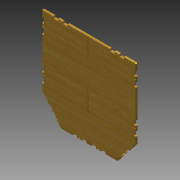
# Autodesk Inventor part: tampa_mdf
Saved by Autodesk Inventor 2014 (Build 180170000, 170)
## iProperties
Created: 2014-11-10
Part Number: tampa_mdf
Material: Generic
Document SubType Name: Modeling
Designer: Gabriel
Density: 1 g/cm^3
Appearance: Default
Author: Gabriel
Autodesk Inventor part; units mm, degrees
ref_plane "YZ Plane" through (0, 0, 0) normal (1, 0, 0) x (0, 1, 0)
ref_plane "XZ Plane" through (0, 0, 0) normal (0, 1, 0) x (-1, 0, 0)
ref_plane "XY Plane" through (0, 0, 0) normal (0, 0, 1) x (1, 0, 0)
sketch "Sketch1" plane through (0, 0, 0) normal (0, 1, 0) x (-1, 0, 0)
  line L0 (0, -150) -> (40, -200)
  line L1 (160, -200) -> (200, -150)
  line L2 (0, -150) -> (0, -120)
  line L3 (0, -150) -> (0, -120)
  line L4 (0, -120) -> (0, -150)
  line L5 (200, -120) -> (200, -150)
  line L6 (40, -200) -> (65, -200)
  line L7 (160, -200) -> (135, -200)
  line L8 (65, -200) -> (40, -200)
  line L9 (200, -120) -> (200, -150)
  line L10 (0, -120) -> (0, 0)
  line L11 (200, 0) -> (200, -120)
  line L12 (0, 0) -> (200, 0)
  line L13 (0, 0) -> (2.5, 0)
  line L14 (65, -200) -> (135, -200)
  line L15 (160, -200) -> (169.9951, -187.5061)
  line L16 (169.9951, -187.5061) -> (189.9854, -162.5183)
  line L17 (189.9854, -162.5183) -> (188.0332, -160.9566)
  circle A0 centre (188.0332, -160.9566) radius 1.5
  circle A1 centre (168.0429, -185.9444) radius 1.5
  line L18 (40, -200) -> (30.0049, -187.5061)
  line L19 (30.0049, -187.5061) -> (31.9571, -185.9444)
  circle A2 centre (31.9571, -185.9444) radius 1.5
  circle A3 centre (11.9668, -160.9566) radius 1.5
  line L20 (40, -200) -> (33.753, -192.1913)
  line L21 (27.5061, -184.3826) -> (21.2591, -176.5739)
  line L22 (0, -150) -> (6.247, -157.8087)
  line L23 (12.4939, -165.6174) -> (18.7409, -173.4261)
  line L24 (160, -200) -> (166.247, -192.1913)
  line L25 (166.247, -192.1913) -> (172.4939, -184.3826)
  line L26 (168.98, -184.7731) -> (168.0429, -185.9444)
  line L27 (200, -150) -> (193.753, -157.8087)
  line L28 (193.753, -157.8087) -> (187.5061, -165.6174)
  line L29 (187.5061, -165.6174) -> (181.2591, -173.4261)
  line L30 (135, -200) -> (135, -195)
  line L31 (135, -195) -> (125, -195)
  line L32 (125, -195) -> (125, -200)
  line L33 (125, -195) -> (115, -195)
  line L34 (115, -195) -> (115, -200)
  line L35 (115, -195) -> (105, -195)
  line L36 (105, -195) -> (105, -200)
  line L37 (40, -200) -> (65, -200)
  line L38 (65, -200) -> (65, -195)
  line L39 (65, -195) -> (75, -195)
  line L40 (75, -195) -> (75, -200)
  line L41 (75, -200) -> (85, -200)
  line L42 (85, -200) -> (85, -195)
  line L43 (85, -195) -> (95, -195)
  line L44 (95, -195) -> (95, -200)
  line L45 (0, -150) -> (0, -105)
  line L46 (0, -95) -> (0, -85)
  line L47 (0, -75) -> (0, -45)
  line L48 (0, -45) -> (5, -45)
  line L49 (5, -45) -> (5, -35)
  line L50 (5, -35) -> (0, -35)
  line L51 (0, -35) -> (0, -25)
  line L52 (0, -25) -> (5, -25)
  line L53 (5, -25) -> (5, -15)
  line L54 (5, -15) -> (0, -15)
  line L55 (0, -45) -> (200, -45)
  line L56 (195, -45) -> (195, -35)
  line L57 (195, -35) -> (200, -35)
  line L58 (0, -25) -> (200, -25)
  line L59 (195, -25) -> (195, -15)
  line L60 (195, -15) -> (200, -15)
  line L61 (0, 0) -> (25, 0)
  line L62 (25, 0) -> (25, -5)
  line L63 (25, -5) -> (35, -5)
  line L64 (35, -5) -> (35, 0)
  line L65 (35, -5) -> (45, -5)
  line L66 (45, -5) -> (45, 0)
  line L67 (45, -5) -> (55, -5)
  line L68 (55, -5) -> (55, 0)
  line L69 (200, 0) -> (175, 0)
  line L70 (175, 0) -> (175, -5)
  line L71 (175, -5) -> (165, -5)
  line L72 (165, -5) -> (165, 0)
  line L73 (165, -5) -> (155, -5)
  line L74 (155, -5) -> (155, 0)
  line L75 (155, -5) -> (145, -5)
  line L76 (145, -5) -> (145, 0)
  line L77 (40, -200) -> (30.0049, -187.5061)
  line L78 (30, -187.5) -> (32.1871, -190.2338)
  line L79 (11.9668, -160.9566) -> (10.0146, -162.5183)
  line L80 (0, -150) -> (10.0146, -162.5183)
  line L81 (10.0146, -162.5183) -> (8.7059, -160.8824)
  line L82 (168.0429, -185.9444) -> (169.9951, -187.5061)
  line L83 (160, -200) -> (169.9951, -187.5061)
  line L84 (169.9951, -187.5061) -> (167.8081, -190.2399)
  line L85 (189.9854, -162.5183) -> (191.2941, -160.8824)
  line L86 (40, -200) -> (39.3753, -199.2191)
  line L87 (30, -187.5) -> (28.4431, -185.5539)
  line L88 (28.4431, -185.5539) -> (30.8818, -183.603)
  line L89 (30.8818, -183.603) -> (24.6348, -175.7943)
  line L90 (24.6348, -175.7943) -> (22.1962, -177.7452)
  line L91 (169.9951, -187.5061) -> (171.5569, -185.5539)
  line L92 (171.5569, -185.5539) -> (169.1182, -183.603)
  line L93 (169.1182, -183.603) -> (175.3652, -175.7943)
  line L94 (175.3652, -175.7943) -> (177.8038, -177.7452)
  line L95 (22.1962, -177.7452) -> (20.5545, -175.6931)
  line L96 (20.5545, -175.6931) -> (22.9931, -173.7422)
  line L97 (22.9931, -173.7422) -> (16.7462, -165.9335)
  line L98 (16.7462, -165.9335) -> (14.3075, -167.8844)
  line L99 (177.8038, -177.7452) -> (179.4455, -175.6931)
  line L100 (179.4455, -175.6931) -> (177.0069, -173.7422)
  line L101 (177.0069, -173.7422) -> (183.2538, -165.9335)
  line L102 (183.2538, -165.9335) -> (185.6925, -167.8844)
  line L103 (0, -45) -> (0, -105)
  line L104 (0, -105) -> (5, -105)
  line L105 (5, -105) -> (5, -115)
  line L106 (5, -115) -> (0, -115)
  line L107 (5, -125) -> (0, -125)
  line L108 (5, -125) -> (5, -135)
  line L109 (5, -135) -> (0, -135)
  line L110 (5, -135) -> (200, -135)
  line L111 (5, -125) -> (200, -125)
  line L112 (5, -115) -> (200, -115)
  line L113 (5, -105) -> (200, -105)
  line L114 (200, -115) -> (195, -115)
  line L115 (195, -115) -> (195, -105)
  line L116 (195, -135) -> (195, -125)
  line L117 (0, -125) -> (0, -120)
  line L118 (0, -120) -> (2.5, -120)
  circle A4 centre (2.5, -120) radius 1.5
  line L119 (200, -120) -> (197.5, -120)
  circle A5 centre (197.5, -120) radius 1.5
  point P0 (200, -95)
  point P1 (200, -85)
  point P2 (200, -75)
  point P3 (33.1284, -191.4104)
  dimension "d293" = 3
  dimension "d2" = 150
  dimension "d6" = 200
  dimension "d26" = 25
  dimension "d37" = 30
  dimension "d41" = 2.5
  dimension "d277" = 120
  dimension "d296" = 16
  dimension "d297" = 32
  dimension "d299" = 3
  dimension "d333" = 10
  dimension "d338" = 10
  dimension "d342" = 10
  dimension "d363" = 5
  dimension "d364" = 10
  dimension "d365" = 10
  dimension "d366" = 10
  dimension "d367" = 25
  dimension "d368" = 5
  dimension "d369" = 10
  dimension "d370" = 10
  dimension "d371" = 10
  dimension "d381" = 5
  dimension "d382" = 10
  dimension "d383" = 10
  dimension "d384" = 5
  dimension "d385" = 10
  dimension "d391" = 25
  dimension "d392" = 5
  dimension "d393" = 10
  dimension "d394" = 10
  dimension "d395" = 10
  dimension "d396" = 25
  dimension "d397" = 5
  dimension "d398" = 10
  dimension "d401" = 10
  dimension "d402" = 10
  dimension "d408" = 2.095
  dimension "d434" = 3.123
  dimension "d435" = 10
  dimension "d436" = 2.5
  dimension "d437" = 2.5
  dimension "d438" = 3.123
  dimension "d439" = 10
  dimension "d440" = 2.628
  dimension "d441" = 3.123
  dimension "d442" = 10
  dimension "d443" = 2.628
  dimension "d444" = 3.123
  dimension "d445" = 10
  dimension "d448" = 20
  dimension "d449" = 60
  dimension "d450" = 5
  dimension "d451" = 10
  dimension "d453" = 10
  dimension "d454" = 10
  dimension "d455" = 5
  dimension "d456" = 10
  dimension "d459" = 5
  dimension "d460" = 2.5
  dimension "d461" = 3
  dimension "d462" = 2.5
  dimension "d463" = 3
  constraints: 232 end point, 41 perpendicular, 38 point on line, 10 parallel, 8 horizontal, 8 vertical, 7 coincident, 5 centre point, 5 collinear, 1 midpoint, 57 other
  measures "d2" distance of L2.start point (0, 0)
  measures "d6" distance of L1.end L2.start
  measures "d26" distance of L1.start L7.end
  measures "d37" distance of L5.start L1.end
  measures "d41" distance of L13.start L13.end
  measures "d277" distance of L1.start L6.start
  measures "d296" distance of L6.start L18.end
  measures "d297" distance of L19.end point (11.967, -160.957)
  measures "d299" diameter of A3
  measures "d333" distance of L6.start L20.end
  measures "d338" distance of L2.start L22.end
  measures "d342" distance of L23.start L23.end
  measures "d363" distance of L7.end L30.end
  measures "d364" distance of L30.end L31.end
  measures "d365" distance of L31.end L33.end
  measures "d366" distance of L33.end L35.end
  measures "d367" distance of L6.start L6.end
  measures "d368" distance of L6.end L38.end
  measures "d369" distance of L38.end L39.end
  measures "d370" distance of L40.end L41.end
  measures "d371" distance of L42.end L43.end
  measures "d381" distance of L47.end L48.end
  measures "d382" distance of L48.end L49.end
  measures "d383" distance of L50.end L51.end
  measures "d384" distance of L51.end L52.end
  measures "d385" distance of L52.end L53.end
  measures "d391" distance of L13.start L61.end
  measures "d392" distance of L61.end L62.end
  measures "d393" distance of L62.end L63.end
  measures "d394" distance of L63.end L65.end
  measures "d395" distance of L65.end L67.end
  measures "d396" distance of L69.start L69.end
  measures "d397" distance of L69.end L70.end
  measures "d398" distance of L70.end L71.end
  measures "d401" distance of L71.end L73.end
  measures "d402" distance of L73.end L75.end
  measures "d408" distance of L79.end L81.end
  measures "d434" distance of L87.end L88.end
  measures "d435" distance of L88.end L89.end
  measures "d436" distance between parallel lines of L88 L19
  measures "d437" distance of L82.end L91.end
  measures "d438" distance of L91.end L92.end
  measures "d439" distance of L92.end L93.end
  measures "d440" distance of L90.end L95.end
  measures "d441" distance of L95.end L96.end
  measures "d442" distance of L96.end L97.end
  measures "d443" distance of L94.end L99.end
  measures "d444" distance of L99.end L100.end
  measures "d445" distance of L100.end L101.end
  measures "d448" distance between parallel lines of L58 L55
  measures "d449" distance of L47.end L103.end
  measures "d450" distance of L103.end L104.end
  measures "d451" distance of L104.end L105.end
  measures "d453" distance of L107.start L108.end
  measures "d454" distance between parallel lines of L107 L106
  measures "d455" distance of L112.end L114.end
  measures "d456" distance between parallel lines of L114 L113
  measures "d459" distance of L107.end L2.end
  measures "d460" distance of L2.end L118.end
  measures "d461" diameter of A4
  measures "d462" distance of L5.start L119.end
  measures "d463" diameter of A5
extrude "Extrusion1" add sketch "Sketch1" along normal blind 5 contours L2 L109 L110 L5 L1 L102 L101 L100 L94 L93 L92 L7 L30 L31 L33 L35 L36 L14 L44 L43 L42 L40 L39 L38 L6 L0 L88 L89 L90 L96 L97 L98 | L2 L107 L108 L109 | L2 L10 L106 L112 L11 L5 L111 L107 | L108 L111 L116 L110 | L116 L111 L5 L110 | L10 L104 L105 L106 | L98 L97 L96 L0 | L10 L48 L55 L11 L113 L104 | L105 L113 L115 L112 | L115 L113 L11 L112 | L90 L89 L88 L0 | L10 L50 L49 L48 | L55 L56 L57 L11 | L10 L52 L58 L11 L57 L56 L55 L49 L50 | L1 L100 L101 L102 | L10 L54 L53 L52 | L58 L59 L60 L11 | L10 L12 L62 L63 L65 L67 L68 L76 L75 L73 L71 L70 L11 L60 L59 L58 L53 L54 | L1 L92 L93 L94 | L70 L71 L72 L12 | L12 L64 L63 L62 | L72 L73 L74 L12 | L12 L66 L65 L64 | L74 L75 L76 L12 | L12 L68 L67 L66 | L38 L39 L40 L14 | L42 L43 L44 L14 | L14 L32 L31 L30 | L14 L34 L33 L32 | L36 L35 L34 L14 | A0 | A1 L82 L26 | L26 L82 A1 | A2 | A3 | A4 | A5
sketch "Sketch2" plane through (0, 0, 0) normal (0, -1, 0) x (1, 0, 0)
  circle A0 centre (-2.5, -30) radius 1
  circle A1 centre (-2.5, -120) radius 1
  circle A2 centre (-2.5, -150) radius 1
  circle A3 centre (-197.5, -30) radius 1
  circle A4 centre (-197.5, -120) radius 1
  circle A5 centre (-197.5, -150) radius 1
  line L0 (-5, 0) -> (-2.5, 0)
  line L1 (0, 0) -> (0, -150) projected
  line L2 (-200, -150) -> (-200, 0) projected
  line L3 (-160, -200) -> (-160, -197.5)
  circle A6 centre (-155, -197.5) radius 1
  circle A7 centre (-120, -197.5) radius 1
  circle A8 centre (-45, -197.5) radius 1
  circle A9 centre (-80, -197.5) radius 1
  line L4 (-200, 0) -> (0, 0) projected
  line L5 (-197.5, -30) -> (-197.5, -2.5)
  line L6 (-197.5, -2.5) -> (-160, -2.5)
  line L7 (-160, -2.5) -> (-120, -2.5)
  line L8 (-120, -2.5) -> (-80, -2.5)
  line L9 (-80, -2.5) -> (-40, -2.5)
  line L10 (-40, -2.5) -> (-2.5, -2.5)
  circle A10 centre (-160, -2.5) radius 1
  circle A11 centre (-120, -2.5) radius 1
  circle A12 centre (-80, -2.5) radius 1
  circle A13 centre (-40, -2.5) radius 1
  circle A14 centre (-2.5, -2.5) radius 1
  circle A15 centre (-197.5, -2.5) radius 1
  line L11 (-120, -2.5) -> (-100, -2.5)
  dimension "d49" = 2
  dimension "d52" = 2
  dimension "d53" = 2
  dimension "d60" = 2
  dimension "d63" = 2
  dimension "d64" = 2
  dimension "d65" = 2.5
  dimension "d66" = 2.5
  dimension "d74" = 30
  dimension "d147" = 2.5
  dimension "d156" = 2
  dimension "d157" = 2
  dimension "d158" = 2
  dimension "d159" = 2
  dimension "d160" = 35
  dimension "d161" = 40
  dimension "d162" = 35
  dimension "d191" = 30
  dimension "d195" = 30
  dimension "d196" = 2.5
  dimension "d199" = 2.5
  dimension "d200" = 2.5
  dimension "d201" = 30
  dimension "d202" = 27.5
  dimension "d203" = 37.5
  dimension "d208" = 2
  dimension "d209" = 2
  dimension "d210" = 2
  dimension "d211" = 2
  dimension "d212" = 2
  dimension "d248" = 2
  dimension "d273" = 40
  dimension "d274" = 40
  dimension "d275" = 40
  dimension "d276" = 37.5
  dimension "d278" = 5
  dimension "d325" = 20
  constraints: 18 end point, 16 centre point, 6 coincident, 4 collinear, 2 perpendicular, 1 midpoint
  measures "d49" diameter of A0
  measures "d52" diameter of A1
  measures "d53" diameter of A2
  measures "d60" diameter of A3
  measures "d63" diameter of A4
  measures "d64" diameter of A5
  measures "d65" distance of L0.start L0.end
  measures "d66" distance of L1.start L0.end
  measures "d74" distance of A2.centre A1.centre
  measures "d147" distance of L3.start L3.end
  measures "d156" diameter of A6
  measures "d157" diameter of A7
  measures "d158" diameter of A8
  measures "d159" diameter of A9
  measures "d160" distance of A7.centre A6.centre
  measures "d161" distance of A9.centre A7.centre
  measures "d162" distance of A8.centre A9.centre
  measures "d191" distance from line of L4 L5.start
  measures "d195" distance of A5.centre A4.centre
  measures "d196" distance from line of L2 L5.start
  measures "d199" distance from line of L2 A4.centre
  measures "d200" distance from line of A1.centre L1
  measures "d201" distance from line of L4 A0.centre
  measures "d202" distance of L5.start L5.end
  measures "d203" distance of L5.end L6.end
  measures "d208" diameter of A10
  measures "d209" diameter of A11
  measures "d210" diameter of A12
  measures "d211" diameter of A13
  measures "d212" diameter of A14
  measures "d248" diameter of A15
  measures "d273" distance of L6.end L7.end
  measures "d274" distance of L7.end L8.end
  measures "d275" distance of L8.end L9.end
  measures "d276" distance of L9.end L10.end
  measures "d278" distance of L3.end A6.centre
  measures "d325" distance of L11.start L11.end
extrude "Extrusion2" cut sketch "Sketch2" against normal blind 5 contours A3
hole "Hole11" at (-120, 0, -197.5) direction (0, 1, 0) diameter 3 end through all
hole "Hole12" at (-80, 0, -197.5) direction (0, 1, 0) diameter 3 end through all
hole "Hole14" at (-160, 0, -2.5) direction (0, 1, 0) diameter 3 end through all
hole "Hole17" at (-40, 0, -2.5) direction (0, 1, 0) diameter 3 end through all
hole "Hole20" at (-197.5, 0, -30) direction (0, 1, 0) diameter 3 end through all
fillet "Fillet8" radius 2 2 edges at (0, 5, -75) (0, 0, -75)
fillet "Fillet9" radius 2 5 edges at (-21, 5, -176.25) (-0.5858, 4.4142, -150.7322) (0, 2.5, -150) (-0.5858, 0.5858, -150.7322) (-21, 0, -176.25)
fillet "Fillet10" radius 2 5 edges at (-40.7502, 4.4142, -200) (-40, 2.5, -200) (-40.7502, 0.5858, -200) (-101.2806, 0, -200) (-101.2806, 5, -200)
fillet "Fillet11" radius 2 5 edges at (-160.4686, 4.4142, -199.4142) (-160, 2.5, -200) (-160.4686, 0.5858, -199.4142) (-180.8, 0, -174) (-180.8, 5, -174)
fillet "Fillet12" radius 2 5 edges at (-200, 4.4142, -149.0623) (-200, 2.5, -150) (-200, 0.5858, -149.0623) (-200, 0, -73.3992) (-200, 5, -73.3992)
fillet "Fillet13" radius 2 8 edges at (-0.5858, 4.4142, 0) (0, 2.5, 0) (-0.5858, 0.5858, 0) (-100, 0, 0) (-199.4142, 0.5858, 0) (-200, 2.5, 0) (-199.4142, 4.4142, 0) (-100, 5, 0)
sketch "Sketch3" plane through (0, 0, 0) normal (0, -1, 0) x (1, 0, 0)
  point P0 (0, 0)
hole "Hole21" at (-2.5, 0, -30) direction (0, 1, 0) diameter 3 end through all
extrude "Extrusion5" cut sketch "Sketch1" along normal blind 5 contours A0
extrude "Extrusion6" cut sketch "Sketch1" along normal blind 5 contours A1 L82 L26 | L26 L82 A1
hole "Hole22" at (-11.9668, 0, -160.9566) direction (0, -1, 0) diameter 3 end through all
hole "Hole23" at (-31.9571, 0, -185.9444) direction (0, 1, 0) diameter 3 end through all
hole "Hole24" at (-11.9668, 0, -160.9566) direction (0, 1, 0) diameter 3 end through all
extrude "Extrusion13" cut sketch "Sketch1" along normal blind 5 contours L38 L39 L40 L14 | L42 L43 L44 L14 | L14 L32 L31 L30 | L36 L35 L34 L14
extrude "Extrusion16" cut sketch "Sketch1" along normal blind 5 contours L70 L71 L72 L12 | L12 L64 L63 L62 | L74 L75 L76 L12 | L12 L68 L67 L66
extrude "Extrusion19" cut sketch "Sketch1" along normal blind 5 contours L98 L97 L96 L0 | L90 L89 L88 L0 | L1 L100 L101 L102 | L1 L92 L93 L94
extrude "Extrusion20" cut sketch "Sketch1" along normal blind 5 contours L2 L107 L108 L109 | L116 L111 L5 L110 | L10 L104 L105 L106 | L115 L113 L11 L112 | L10 L50 L49 L48 | L55 L56 L57 L11 | L10 L54 L53 L52 | L58 L59 L60 L11
hole "Hole25" at (-2.5, 0, -120) direction (0, 1, 0) diameter 3 end through all
hole "Hole26" at (-197.5, 0, -120) direction (0, 1, 0) diameter 3 end through all
body "Solid1"
